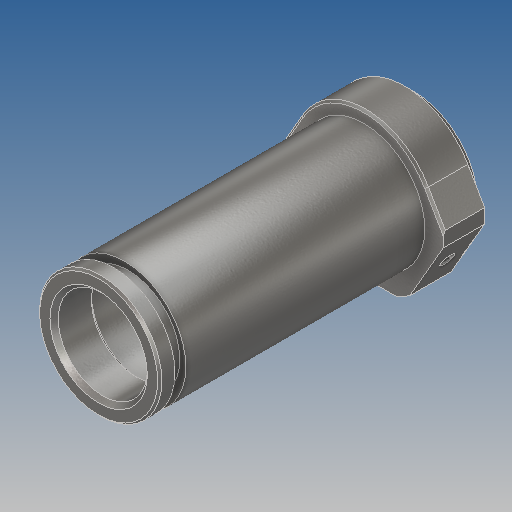
# Autodesk Inventor part: piston_reservoir
Saved by Autodesk Inventor 2019 (Build 230136000, 136)
## iProperties
Created: 2019-03-25
Part Number: piston_reservoir
Material: Acier, galvanisé
Document SubType Name: Modeling
Designer: theor
Density: 7.85 g/cm^3
Appearance: Galvanisé
Mass: 181.554 g
Surface Area: 151.415 cm^2
Volume: 23.1278 cm^3
Author: theor
Autodesk Inventor part; units mm, degrees
ref_plane "YZ Plane" through (0, 0, 0) normal (1, 0, 0) x (0, 1, 0)
ref_plane "XZ Plane" through (0, 0, 0) normal (0, 1, 0) x (-1, 0, 0)
sketch "Esquisse1" plane through (0, 0, 0) normal (1, 0, 0) x (0, 1, 0)
  line L0 (0, 0) -> (0, 68.1349)
  line L1 (14.75, 69.6949) -> (14.75, 12)
  line L2 (15.5, 0) -> (4, 0)
  line L3 (4, 0) -> (4, 4)
  line L4 (4, 4) -> (9.25, 4)
  line L5 (14.75, 76) -> (10.75, 76)
  line L6 (14.75, 12) -> (17.5, 12)
  line L7 (17.5, 12) -> (17.5, 2)
  line L8 (17.5, 2) -> (15.5, 0)
  line L9 (12.25, 12) -> (9.25, 9)
  line L10 (9.25, 9) -> (9.25, 4)
  line L11 (10.75, 76) -> (10.75, 66)
  line L12 (10.75, 66) -> (12.25, 66)
  line L13 (12.25, 66) -> (12.25, 12)
  line L14 (14.75, 76) -> (14.75, 72.3051)
  line L15 (14.75, 72.3051) -> (12.45, 73.1422)
  line L16 (12.45, 73.1422) -> (12.45, 68.8578)
  line L17 (12.45, 68.8578) -> (14.75, 69.6949)
  circle A0 centre (13.95, 71) radius 1.5 construction
  dimension "d1" = 29.5
  dimension "d2" = 8
  dimension "d3" = 4
  dimension "d6" = 2
  dimension "d7" = 2
  dimension "d8" = 10
  dimension "d26" = 3
  dimension "d27" = 3
  dimension "d31" = 2.5
  dimension "d32" = 4
  dimension "d34" = 10
  dimension "d35" = 64
  dimension "d36" = 70
  dimension "d37" = 70
  dimension "d38" = 3
  dimension "d39" = 0.8
  dimension "d40" = 5
  dimension "d47" = 35
  constraints: 36 end point, 9 vertical, 5 horizontal, 3 tangent, 2 horizontal alignment, 1 centre point, 1 collinear
  measures "d1" diameter of L1 L0
  measures "d2" diameter of L3 L0
  measures "d3" distance of L2.end L3.end
  measures "d6" horizontal distance of L7.end L2.start
  measures "d7" horizontal distance of L7.end L2.start
  measures "d8" distance of L6.end L7.end
  measures "d26" horizontal distance of L9.start L9.end
  measures "d27" horizontal distance of L9.start L9.end
  measures "d31" distance between parallel lines of L13 L1
  measures "d32" distance between parallel lines of L1 L11
  measures "d34" distance from line of L5 L11.end
  measures "d35" distance between parallel lines of L6 L5
  measures "d36" angle of L16 L17
  measures "d37" angle of L16 L15
  measures "d38" diameter of A0
  measures "d39" distance from line of L1 A0.centre
  measures "d40" vertical distance of L5.end A0.centre
  measures "d47" diameter of L7 L0
revolve "Révolution1" add sketch "Esquisse1" angle 360 about axis through (0, 0, 0) along (0, 0, 1)
ref_plane "Plan de construction1" through (0, 0, 2) normal (0, 0, -1) x (-1, 0, 0)
sketch "Esquisse3" plane through (0, 0, 2) normal (0, 0, -1) x (-1, 0, 0)
  line L0 (10.1036, 17.5) -> (20.2073, 0)
  line L1 (20.2073, 0) -> (10.1036, -17.5)
  line L2 (10.1036, -17.5) -> (-10.1036, -17.5)
  line L3 (-10.1036, -17.5) -> (-20.2073, 0)
  line L4 (-20.2073, 0) -> (-10.1036, 17.5)
  line L5 (-10.1036, 17.5) -> (10.1036, 17.5)
  circle A0 centre (0, 0) radius 17.5 projected
  line L6 (15.1554, 8.75) -> (-15.1554, 8.75)
  arc A1 (-15.1554, 8.75) -> (15.1554, 8.75) centre (0, 0) ccw
  constraints: 14 end point, 2 coincident, 2 midpoint, 2 point on circle, 1 centre point, 1 horizontal, 1 tangent, 13 other
extrude "Extrusion1" add sketch "Esquisse3" against normal blind 10 contours L0 L1 A0 | A0 L3 L4 | L1 L2 A0 | A0 L2 L3
chamfer "Chanfrein1" distance 2 angle 45 1 edges at (0, -9.25, 4)
chamfer "Chanfrein2" distance 2 angle 45 4 edges at (-20.2073, 0, 7) (-10.1036, -17.5, 7) (10.1036, -17.5, 7) (20.2073, 0, 7)
sketch "Esquisse4" plane through (-8.1036, -17.5, 2) normal (0, -1, 0) x (1, 0, 0)
  line L0 (16.2073, 10) -> (16.2073, 0) projected
  line L1 (0, 10) -> (16.2073, 10) projected
  line L2 (0, 0) -> (0, 10) projected
  line L3 (8.1036, 0) -> (0, 0) projected
  line L4 (16.2073, 0) -> (8.1036, 0) projected
  point P0 (8.1036, -2)
  point P1 (8.1036, 5)
  point P2 (16.2073, 5)
  constraints: 1 horizontal alignment, 1 midpoint, 1 vertical alignment
hole "Perçage1" at (0, -17.5, 7) direction (0, 1, 0) diameter 3.242 depth 6 tip angle 118 thread size "M4x0.7" class "6H" standard "ISO Metric profile"
chamfer "Chanfrein3" distance 1 angle 45 2 edges at (0, -10.75, 76) (0, -10.75, 66)
pattern_circular "Réseau circulaire1" count 3 over 120 about axis through (0, 0, -10) along (0, 0, 1) of "Perçage1" both ways yes
chamfer "Chanfrein4" distance 0.5 angle 45 3 edges at (0, 17.5, 12) (17.1814, 5.241, 12) (-17.1814, 5.241, 12)
chamfer "Chanfrein5" distance 0.5 angle 45 1 edges at (0, -14.75, 76)
equation "\"d7\" = d6"
equation "\"d27\" = d26"
equation "\"d37\" = d36"
